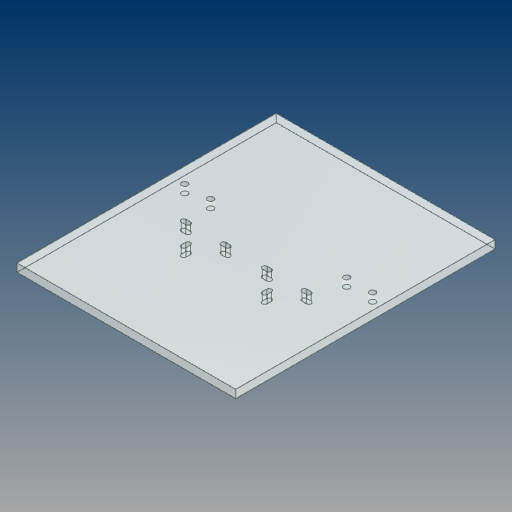
# Autodesk Inventor part: 12_Tam_go_top
Saved by Autodesk Inventor 2021 (Build 250183000, 183)
## iProperties
Created: 2024-04-09
Part Number: 12_Tam_go_top
Material: Glass
Document SubType Name: Modeling
Designer: Admin
Density: 2.18 g/cm^3
Appearance: Clear
Mass: 1871.55 g
Surface Area: 1862.48 cm^2
Volume: 858.509 cm^3
Author: Admin
Autodesk Inventor part; units mm, degrees
ref_plane "YZ Plane" through (0, 0, 0) normal (1, 0, 0) x (0, 1, 0)
ref_plane "XZ Plane" through (0, 0, 0) normal (0, 1, 0) x (-1, 0, 0)
ref_plane "XY Plane" through (0, 0, 0) normal (0, 0, 1) x (1, 0, 0)
sketch "Sketch1" plane through (0, 0, 0) normal (0, 1, 0) x (-1, 0, 0)
  line L0 (-135, 160) -> (135, 160)
  line L1 (135, 160) -> (135, -160)
  line L2 (135, -160) -> (-135, -160)
  line L3 (-135, -160) -> (-135, 160)
  line L4 (-135, 160) -> (135, -160) construction
  line L5 (135, 160) -> (-135, -160) construction
  point P0 (0, 0)
  dimension "d0" = 270
  dimension "d1" = 320
  constraints: 12 end point, 2 midpoint, 2 parallel, 1 horizontal, 1 perpendicular
  measures "d0" distance of L1.end L2.end
  measures "d1" distance between parallel lines of L0 L2
extrude "Extrusion1" add sketch "Sketch1" along normal blind 10
sketch "Sketch2" plane through (0, 10, 0) normal (0, 1, 0) x (1, 0, 0)
  line L0 (57, -25.5) -> (57, -50) projected
  line L1 (57, -25.5) -> (43, -25.5) projected
  line L2 (43, -50) -> (43, -25.5) projected
  line L3 (57, -50) -> (43, -50) projected
  arc A0 (53, -33.75) -> (47, -33.75) centre (50, -33.75) ccw projected
  line L4 (53, -39.25) -> (53, -33.75) projected
  arc A1 (47, -39.25) -> (53, -39.25) centre (50, -39.25) ccw projected
  line L5 (47, -33.75) -> (47, -39.25) projected
  line L6 (63.5, -5) -> (88, -5) projected
  line L7 (63.5, -5) -> (63.5, -19) projected
  line L8 (88, -19) -> (63.5, -19) projected
  line L9 (88, -5) -> (88, -19) projected
  arc A2 (71.75, -9) -> (71.75, -15) centre (71.75, -12) ccw projected
  line L10 (77.25, -9) -> (71.75, -9) projected
  arc A3 (77.25, -15) -> (77.25, -9) centre (77.25, -12) ccw projected
  line L11 (71.75, -15) -> (77.25, -15) projected
  line L12 (36.5, -19) -> (12, -19) projected
  line L13 (36.5, -19) -> (36.5, -5) projected
  line L14 (12, -5) -> (36.5, -5) projected
  line L15 (12, -19) -> (12, -5) projected
  arc A4 (28.25, -15) -> (28.25, -9) centre (28.25, -12) ccw projected
  line L16 (22.75, -15) -> (28.25, -15) projected
  arc A5 (22.75, -9) -> (22.75, -15) centre (22.75, -12) ccw projected
  line L17 (28.25, -9) -> (22.75, -9) projected
  line L18 (-36.5, -5) -> (-12, -5) projected
  line L19 (-36.5, -5) -> (-36.5, -19) projected
  line L20 (-12, -19) -> (-36.5, -19) projected
  line L21 (-12, -5) -> (-12, -19) projected
  arc A6 (-28.25, -9) -> (-28.25, -15) centre (-28.25, -12) ccw projected
  line L22 (-22.75, -9) -> (-28.25, -9) projected
  arc A7 (-22.75, -15) -> (-22.75, -9) centre (-22.75, -12) ccw projected
  line L23 (-28.25, -15) -> (-22.75, -15) projected
  line L24 (-43, -25.5) -> (-43, -50) projected
  line L25 (-43, -25.5) -> (-57, -25.5) projected
  line L26 (-57, -50) -> (-57, -25.5) projected
  line L27 (-43, -50) -> (-57, -50) projected
  arc A8 (-47, -33.75) -> (-53, -33.75) centre (-50, -33.75) ccw projected
  line L28 (-47, -39.25) -> (-47, -33.75) projected
  arc A9 (-53, -39.25) -> (-47, -39.25) centre (-50, -39.25) ccw projected
  line L29 (-53, -33.75) -> (-53, -39.25) projected
  line L30 (-63.5, -19) -> (-88, -19) projected
  line L31 (-63.5, -19) -> (-63.5, -5) projected
  line L32 (-88, -5) -> (-63.5, -5) projected
  line L33 (-88, -19) -> (-88, -5) projected
  arc A10 (-71.75, -15) -> (-71.75, -9) centre (-71.75, -12) ccw projected
  line L34 (-77.25, -15) -> (-71.75, -15) projected
  arc A11 (-77.25, -9) -> (-77.25, -15) centre (-77.25, -12) ccw projected
  line L35 (-71.75, -9) -> (-77.25, -9) projected
  line L36 (-108.92, 42.1) -> (-108.92, 39.2309) projected
  line L37 (-108.52, 39) -> (-108.92, 39.2309) projected
  line L38 (-108.92, 38.7691) -> (-108.52, 39) projected
  line L39 (-108.92, 38.7691) -> (-108.92, 35.0867) projected
  line L40 (-108.92, 35.0867) -> (-117.2017, 32.9363) projected
  arc A12 (-117.2017, 32.9363) -> (-117.2017, 23.0637) centre (-115.92, 28) ccw projected
  line L41 (-117.2017, 23.0637) -> (-101.7351, 19.0476) projected
  arc A13 (-101.7351, 19.0476) -> (-100.579, 18.9) centre (-100.579, 23.5) ccw projected
  line L42 (-100.579, 18.9) -> (-99.2609, 18.9) projected
  arc A14 (-99.2609, 18.9) -> (-98.1048, 19.0476) centre (-99.2609, 23.5) ccw projected
  line L43 (-98.1048, 19.0476) -> (-82.6382, 23.0637) projected
  arc A15 (-82.6382, 23.0637) -> (-82.6382, 32.9363) centre (-83.92, 28) ccw projected
  line L44 (-82.6382, 32.9363) -> (-90.92, 35.0867) projected
  line L45 (-90.92, 42.1) -> (-90.92, 35.0867) projected
  line L46 (-90.92, 42.1) -> (-99.195, 42.1) projected
  line L47 (-99.195, 32.3399) -> (-99.195, 42.1) projected
  arc A16 (-100.645, 32.3399) -> (-99.195, 32.3399) centre (-99.92, 28) ccw projected
  line L48 (-100.645, 32.3399) -> (-100.645, 42.1) projected
  line L49 (-100.645, 42.1) -> (-108.92, 42.1) projected
  circle A17 centre (-115.92, 28) radius 3.8 projected
  circle A18 centre (-83.92, 28) radius 3.8 projected
  line L50 (90.92, 42.1) -> (90.92, 39.2309) projected
  line L51 (91.32, 39) -> (90.92, 39.2309) projected
  line L52 (90.92, 38.7691) -> (91.32, 39) projected
  line L53 (90.92, 38.7691) -> (90.92, 35.0867) projected
  line L54 (90.92, 35.0867) -> (82.6382, 32.9363) projected
  arc A19 (82.6382, 32.9363) -> (82.6382, 23.0637) centre (83.92, 28) ccw projected
  line L55 (82.6382, 23.0637) -> (98.1048, 19.0476) projected
  arc A20 (98.1048, 19.0476) -> (99.2609, 18.9) centre (99.2609, 23.5) ccw projected
  line L56 (99.2609, 18.9) -> (100.579, 18.9) projected
  arc A21 (100.579, 18.9) -> (101.7351, 19.0476) centre (100.579, 23.5) ccw projected
  line L57 (101.7351, 19.0476) -> (117.2017, 23.0637) projected
  arc A22 (117.2017, 23.0637) -> (117.2017, 32.9363) centre (115.92, 28) ccw projected
  line L58 (117.2017, 32.9363) -> (108.92, 35.0867) projected
  line L59 (108.92, 42.1) -> (108.92, 35.0867) projected
  line L60 (108.92, 42.1) -> (100.645, 42.1) projected
  line L61 (100.645, 32.3399) -> (100.645, 42.1) projected
  arc A23 (99.195, 32.3399) -> (100.645, 32.3399) centre (99.92, 28) ccw projected
  line L62 (99.195, 32.3399) -> (99.195, 42.1) projected
  line L63 (99.195, 42.1) -> (90.92, 42.1) projected
  circle A24 centre (83.92, 28) radius 3.8 projected
  circle A25 centre (115.92, 28) radius 3.8 projected
  point P0 (0, 0)
extrude "Extrusion2" cut sketch "Sketch2" against normal blind 10 contours L4 A1 L5 A0 | L10 A3 L11 A2 | L16 A5 L17 A4 | L22 A7 L23 A6 | L28 A9 L29 A8 | L34 A11 L35 A10 | A17 | A18 | A24 | A25
body "Solid1"
